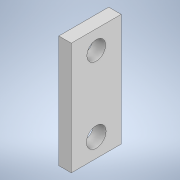
# Autodesk Inventor part: holder
Saved by Autodesk Inventor 2021 (Build 250183000, 183)
## iProperties
Created: 2021-07-14
Part Number: holder
Material: Generic
Document SubType Name: Modeling
Designer: HP
Density: 1 g/cm^3
Appearance: Default
Author: HP
Autodesk Inventor part; units mm, degrees
ref_plane "YZ Plane" through (0, 0, 0) normal (1, 0, 0) x (0, 1, 0)
ref_plane "XZ Plane" through (0, 0, 0) normal (0, 1, 0) x (-1, 0, 0)
ref_plane "XY Plane" through (0, 0, 0) normal (0, 0, 1) x (1, 0, 0)
sketch "Sketch1" plane through (0, 0, 0) normal (1, 0, 0) x (0, 1, 0)
  line L0 (0, 0) -> (90, 0)
  line L1 (90, 0) -> (90, -40)
  line L2 (90, -40) -> (0, -40)
  line L3 (0, -40) -> (0, 0)
  dimension "d0" = 90
  dimension "d1" = 40
  constraints: 8 end point, 2 parallel, 1 horizontal, 1 perpendicular
  measures "d0" distance of L1.end L2.end
  measures "d1" distance of L0.end L1.end
extrude "Extrusion1" add sketch "Sketch1" along normal blind 10
sketch "Sketch2" plane through (0, 0, 0) normal (-1, 0, 0) x (0, 0, 1)
  circle A0 centre (-20, 15) radius 7.8823
  line L0 (0, 0) -> (-40, 0) projected
  dimension "d4" = 15
  constraints: 1 centre point
  measures "d4" distance from line of A0.centre L0
extrude "Extrusion2" cut sketch "Sketch2" against normal mid plane 50
sketch "Sketch3" plane through (0, 0, 0) normal (-1, 0, 0) x (0, 0, 1)
  circle A0 centre (-20, 75) radius 7.5
  line L0 (-40, 90) -> (0, 90) projected
  point P0 (0, 0)
  dimension "d7" = 15
  dimension "d8" = 15
  constraints: 1 centre point
  measures "d7" diameter of A0
  measures "d8" distance from line of L0 A0.centre
extrude "Extrusion3" cut sketch "Sketch3" against normal mid plane 50
body "Solid1"
